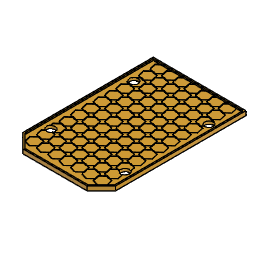
back_cover (Autodesk Fusion 360 design; units mm, degrees)
Autodesk Fusion 360 part; units mm, degrees
(part 1 of 2)
sketch "Sketch1" plane through (0, 0, 0) normal (0, 0, 1) x (1, 0, 0)
  line L0 (0, -30) -> (65.3008, -30)
  line L1 (65.3008, -30) -> (65.3008, 62.8304)
  line L2 (65.3008, 62.8304) -> (0, 62.8304)
  line L3 (0, 62.8304) -> (0, -30)
  line L4 (0, -30) -> (10, -40)
  line L5 (10, -40) -> (55.2691, -40)
  line L6 (55.2691, -40) -> (65.3008, -30)
  constraint horizontal L0
  constraint vertical L1
  constraint horizontal L2
  constraint vertical L3
  constraint perpendicular L3 L5
extrude "Extrude1" add sketch "Sketch1" against normal blind 2
sketch "Sketch2" plane through (0, 0, -2) normal (0, 0, -1) x (1, 0, 0)
  line L0 (65.3008, 30) -> (55.2691, 40)
  line L1 (55.2691, 40) -> (10, 40)
  line L2 (10, 40) -> (0, 30)
  line L3 (0, 30) -> (0, -62.8304)
  line L4 (0, -62.8304) -> (65.3008, -62.8304)
  line L5 (65.3008, -62.8304) -> (65.3008, 30)
  circle A0 centre (6.5514, 16.7159) radius 3
  circle A1 centre (6.5755, -41.7346) radius 3
  circle A2 centre (59.3355, -41.7346) radius 3
  circle A3 centre (58.8128, 16.7193) radius 3
extrude "Extrude2" cut sketch "Sketch2" against normal blind 2 contours A0 | A1 | A2 | A3
fillet "Fillet1" radius 1 3 edges at (0, 62.8304, -1) (65.3008, 62.8304, -1) (32.6504, 62.8304, 0)
sketch "Sketch3" plane through (0, 0, 0) normal (0, 0, 1) x (-1, 0, 0)
  line L0 (-65.3008, -61.8304) -> (0, -61.8304)
  line L1 (0, -61.8304) -> (0, 30)
  line L2 (0, 30) -> (-10, 40)
  line L3 (-10, 40) -> (-55.2691, 40)
  line L4 (-55.2691, 40) -> (-65.3008, 30)
  line L5 (-65.3008, 30) -> (-65.3008, -61.8304)
  circle A0 centre (-6.5514, 16.7159) radius 3
  circle A1 centre (-6.5755, -41.7346) radius 3
  circle A2 centre (-58.8128, 16.7193) radius 3
  circle A3 centre (-59.3355, -41.7346) radius 3
  line L6 (0, -61.8304) -> (0, 30)
  line L7 (0, 30) -> (-10, 40)
  line L8 (-10, 40) -> (-55.2691, 40)
  line L9 (-55.2691, 40) -> (-65.3008, 30)
  line L10 (-65.3008, 30) -> (-65.3008, -61.8304)
  line L11 (0, -61.8304) -> (-65.3008, -61.8304)
  line L12 (-1, -60.8304) -> (-1, 29.5858)
  line L13 (-1, 29.5858) -> (-10.4142, 39)
  line L14 (-10.4142, 39) -> (-54.8558, 39)
  line L15 (-54.8558, 39) -> (-64.3008, 29.5849)
  line L16 (-64.3008, 29.5849) -> (-64.3008, -60.8304)
  line L17 (-64.3008, -60.8304) -> (-1, -60.8304)
  dimension "d111" = -1
extrude "Extrude3" add sketch "Sketch3" along normal blind 1 contours L0 L1 L2 L3 L4 L5 L6 L7 L8 L9 L10 L11
sketch "Sketch4" plane through (0, 0, 0) normal (0, 0, 1) x (1, 0, 0)
  line L0 (36.6966, 8.433) -> (35.7081, 12.9448)
  line L1 (35.7081, 12.9448) -> (31.3065, 14.3446)
  line L2 (31.3065, 14.3446) -> (27.8935, 11.2327)
  line L3 (27.8935, 11.2327) -> (28.8819, 6.7209)
  line L4 (28.8819, 6.7209) -> (33.2835, 5.321)
  line L5 (33.2835, 5.321) -> (36.6966, 8.433)
  line L6 (11.7081, -27.0552) -> (7.3065, -25.6554)
  line L7 (12.6966, -31.567) -> (11.7081, -27.0552)
  line L8 (9.2835, -34.679) -> (12.6966, -31.567)
  line L9 (4.8819, -33.2791) -> (9.2835, -34.679)
  line L10 (3.8935, -28.7673) -> (4.8819, -33.2791)
  line L11 (7.3065, -25.6554) -> (3.8935, -28.7673)
  line L12 (19.7081, -27.0552) -> (15.3065, -25.6554)
  line L13 (20.6966, -31.567) -> (19.7081, -27.0552)
  line L14 (17.2835, -34.679) -> (20.6966, -31.567)
  line L15 (12.8819, -33.2791) -> (17.2835, -34.679)
  line L16 (11.8935, -28.7673) -> (12.8819, -33.2791)
  line L17 (15.3065, -25.6554) -> (11.8935, -28.7673)
  line L18 (27.7081, -27.0552) -> (23.3065, -25.6554)
  line L19 (28.6966, -31.567) -> (27.7081, -27.0552)
  line L20 (25.2835, -34.679) -> (28.6966, -31.567)
  line L21 (20.8819, -33.2791) -> (25.2835, -34.679)
  line L22 (19.8935, -28.7673) -> (20.8819, -33.2791)
  line L23 (23.3065, -25.6554) -> (19.8935, -28.7673)
  line L24 (35.7081, -27.0552) -> (31.3065, -25.6554)
  line L25 (36.6966, -31.567) -> (35.7081, -27.0552)
  line L26 (33.2835, -34.679) -> (36.6966, -31.567)
  line L27 (28.8819, -33.2791) -> (33.2835, -34.679)
  line L28 (27.8935, -28.7673) -> (28.8819, -33.2791)
  line L29 (31.3065, -25.6554) -> (27.8935, -28.7673)
  line L30 (43.7081, -27.0552) -> (39.3065, -25.6554)
  line L31 (44.6966, -31.567) -> (43.7081, -27.0552)
  line L32 (41.2835, -34.679) -> (44.6966, -31.567)
  line L33 (36.8819, -33.2791) -> (41.2835, -34.679)
  line L34 (35.8935, -28.7673) -> (36.8819, -33.2791)
  line L35 (39.3065, -25.6554) -> (35.8935, -28.7673)
  line L36 (51.7081, -27.0552) -> (47.3065, -25.6554)
  line L37 (52.6966, -31.567) -> (51.7081, -27.0552)
  line L38 (49.2835, -34.679) -> (52.6966, -31.567)
  line L39 (44.8819, -33.2791) -> (49.2835, -34.679)
  line L40 (43.8935, -28.7673) -> (44.8819, -33.2791)
  line L41 (47.3065, -25.6554) -> (43.8935, -28.7673)
  line L42 (59.7081, -27.0552) -> (55.3065, -25.6554)
  line L43 (60.6966, -31.567) -> (59.7081, -27.0552)
  line L44 (57.2835, -34.679) -> (60.6966, -31.567)
  line L45 (52.8819, -33.2791) -> (57.2835, -34.679)
  line L46 (51.8935, -28.7673) -> (52.8819, -33.2791)
  line L47 (55.3065, -25.6554) -> (51.8935, -28.7673)
  line L48 (11.7081, -19.0552) -> (7.3065, -17.6554)
  line L49 (12.6966, -23.567) -> (11.7081, -19.0552)
  line L50 (9.2835, -26.679) -> (12.6966, -23.567)
  line L51 (4.8819, -25.2791) -> (9.2835, -26.679)
  line L52 (3.8935, -20.7673) -> (4.8819, -25.2791)
  line L53 (7.3065, -17.6554) -> (3.8935, -20.7673)
  line L54 (19.7081, -19.0552) -> (15.3065, -17.6554)
  line L55 (20.6966, -23.567) -> (19.7081, -19.0552)
  line L56 (17.2835, -26.679) -> (20.6966, -23.567)
  line L57 (12.8819, -25.2791) -> (17.2835, -26.679)
  line L58 (11.8935, -20.7673) -> (12.8819, -25.2791)
  line L59 (15.3065, -17.6554) -> (11.8935, -20.7673)
  line L60 (27.7081, -19.0552) -> (23.3065, -17.6554)
  line L61 (28.6966, -23.567) -> (27.7081, -19.0552)
  line L62 (25.2835, -26.679) -> (28.6966, -23.567)
  line L63 (20.8819, -25.2791) -> (25.2835, -26.679)
  line L64 (19.8935, -20.7673) -> (20.8819, -25.2791)
  line L65 (23.3065, -17.6554) -> (19.8935, -20.7673)
  line L66 (35.7081, -19.0552) -> (31.3065, -17.6554)
  line L67 (36.6966, -23.567) -> (35.7081, -19.0552)
  line L68 (33.2835, -26.679) -> (36.6966, -23.567)
  line L69 (28.8819, -25.2791) -> (33.2835, -26.679)
  line L70 (27.8935, -20.7673) -> (28.8819, -25.2791)
  line L71 (31.3065, -17.6554) -> (27.8935, -20.7673)
  line L72 (43.7081, -19.0552) -> (39.3065, -17.6554)
  line L73 (44.6966, -23.567) -> (43.7081, -19.0552)
  line L74 (41.2835, -26.679) -> (44.6966, -23.567)
  line L75 (36.8819, -25.2791) -> (41.2835, -26.679)
  line L76 (35.8935, -20.7673) -> (36.8819, -25.2791)
  line L77 (39.3065, -17.6554) -> (35.8935, -20.7673)
  line L78 (51.7081, -19.0552) -> (47.3065, -17.6554)
  line L79 (52.6966, -23.567) -> (51.7081, -19.0552)
  line L80 (49.2835, -26.679) -> (52.6966, -23.567)
  line L81 (44.8819, -25.2791) -> (49.2835, -26.679)
  line L82 (43.8935, -20.7673) -> (44.8819, -25.2791)
  line L83 (47.3065, -17.6554) -> (43.8935, -20.7673)
  line L84 (59.7081, -19.0552) -> (55.3065, -17.6554)
  line L85 (60.6966, -23.567) -> (59.7081, -19.0552)
  line L86 (57.2835, -26.679) -> (60.6966, -23.567)
  line L87 (52.8819, -25.2791) -> (57.2835, -26.679)
  line L88 (51.8935, -20.7673) -> (52.8819, -25.2791)
  line L89 (55.3065, -17.6554) -> (51.8935, -20.7673)
  line L90 (11.7081, -11.0552) -> (7.3065, -9.6554)
  line L91 (12.6966, -15.567) -> (11.7081, -11.0552)
  line L92 (9.2835, -18.679) -> (12.6966, -15.567)
  line L93 (4.8819, -17.2791) -> (9.2835, -18.679)
  line L94 (3.8935, -12.7673) -> (4.8819, -17.2791)
  line L95 (7.3065, -9.6554) -> (3.8935, -12.7673)
  line L96 (19.7081, -11.0552) -> (15.3065, -9.6554)
  line L97 (20.6966, -15.567) -> (19.7081, -11.0552)
  line L98 (17.2835, -18.679) -> (20.6966, -15.567)
  line L99 (12.8819, -17.2791) -> (17.2835, -18.679)
  line L100 (11.8935, -12.7673) -> (12.8819, -17.2791)
  line L101 (15.3065, -9.6554) -> (11.8935, -12.7673)
  line L102 (27.7081, -11.0552) -> (23.3065, -9.6554)
  line L103 (28.6966, -15.567) -> (27.7081, -11.0552)
  line L104 (25.2835, -18.679) -> (28.6966, -15.567)
  line L105 (20.8819, -17.2791) -> (25.2835, -18.679)
  line L106 (19.8935, -12.7673) -> (20.8819, -17.2791)
  line L107 (23.3065, -9.6554) -> (19.8935, -12.7673)
  line L108 (35.7081, -11.0552) -> (31.3065, -9.6554)
  line L109 (36.6966, -15.567) -> (35.7081, -11.0552)
  line L110 (33.2835, -18.679) -> (36.6966, -15.567)
  line L111 (28.8819, -17.2791) -> (33.2835, -18.679)
  line L112 (27.8935, -12.7673) -> (28.8819, -17.2791)
  line L113 (31.3065, -9.6554) -> (27.8935, -12.7673)
  line L114 (43.7081, -11.0552) -> (39.3065, -9.6554)
  line L115 (44.6966, -15.567) -> (43.7081, -11.0552)
  line L116 (41.2835, -18.679) -> (44.6966, -15.567)
  line L117 (36.8819, -17.2791) -> (41.2835, -18.679)
  line L118 (35.8935, -12.7673) -> (36.8819, -17.2791)
  line L119 (39.3065, -9.6554) -> (35.8935, -12.7673)
  line L120 (51.7081, -11.0552) -> (47.3065, -9.6554)
  line L121 (52.6966, -15.567) -> (51.7081, -11.0552)
  line L122 (49.2835, -18.679) -> (52.6966, -15.567)
  line L123 (44.8819, -17.2791) -> (49.2835, -18.679)
  line L124 (43.8935, -12.7673) -> (44.8819, -17.2791)
  line L125 (47.3065, -9.6554) -> (43.8935, -12.7673)
  line L126 (59.7081, -11.0552) -> (55.3065, -9.6554)
  line L127 (60.6966, -15.567) -> (59.7081, -11.0552)
  line L128 (57.2835, -18.679) -> (60.6966, -15.567)
  line L129 (52.8819, -17.2791) -> (57.2835, -18.679)
  line L130 (51.8935, -12.7673) -> (52.8819, -17.2791)
  line L131 (55.3065, -9.6554) -> (51.8935, -12.7673)
  line L132 (11.7081, -3.0552) -> (7.3065, -1.6554)
  line L133 (12.6966, -7.567) -> (11.7081, -3.0552)
  line L134 (9.2835, -10.679) -> (12.6966, -7.567)
  line L135 (4.8819, -9.2791) -> (9.2835, -10.679)
  line L136 (3.8935, -4.7673) -> (4.8819, -9.2791)
  line L137 (7.3065, -1.6554) -> (3.8935, -4.7673)
  line L138 (19.7081, -3.0552) -> (15.3065, -1.6554)
  line L139 (20.6966, -7.567) -> (19.7081, -3.0552)
  line L140 (17.2835, -10.679) -> (20.6966, -7.567)
  line L141 (12.8819, -9.2791) -> (17.2835, -10.679)
  line L142 (11.8935, -4.7673) -> (12.8819, -9.2791)
  line L143 (15.3065, -1.6554) -> (11.8935, -4.7673)
  line L144 (27.7081, -3.0552) -> (23.3065, -1.6554)
  line L145 (28.6966, -7.567) -> (27.7081, -3.0552)
  line L146 (25.2835, -10.679) -> (28.6966, -7.567)
  line L147 (20.8819, -9.2791) -> (25.2835, -10.679)
  line L148 (19.8935, -4.7673) -> (20.8819, -9.2791)
  line L149 (23.3065, -1.6554) -> (19.8935, -4.7673)
  line L150 (35.7081, -3.0552) -> (31.3065, -1.6554)
  line L151 (36.6966, -7.567) -> (35.7081, -3.0552)
  line L152 (33.2835, -10.679) -> (36.6966, -7.567)
  line L153 (28.8819, -9.2791) -> (33.2835, -10.679)
  line L154 (27.8935, -4.7673) -> (28.8819, -9.2791)
  line L155 (31.3065, -1.6554) -> (27.8935, -4.7673)
  line L156 (43.7081, -3.0552) -> (39.3065, -1.6554)
  line L157 (44.6966, -7.567) -> (43.7081, -3.0552)
  line L158 (41.2835, -10.679) -> (44.6966, -7.567)
  line L159 (36.8819, -9.2791) -> (41.2835, -10.679)
  line L160 (35.8935, -4.7673) -> (36.8819, -9.2791)
  line L161 (39.3065, -1.6554) -> (35.8935, -4.7673)
  line L162 (51.7081, -3.0552) -> (47.3065, -1.6554)
  line L163 (52.6966, -7.567) -> (51.7081, -3.0552)
  line L164 (49.2835, -10.679) -> (52.6966, -7.567)
  line L165 (44.8819, -9.2791) -> (49.2835, -10.679)
  line L166 (43.8935, -4.7673) -> (44.8819, -9.2791)
  line L167 (47.3065, -1.6554) -> (43.8935, -4.7673)
  line L168 (59.7081, -3.0552) -> (55.3065, -1.6554)
  line L169 (60.6966, -7.567) -> (59.7081, -3.0552)
  line L170 (57.2835, -10.679) -> (60.6966, -7.567)
  line L171 (52.8819, -9.2791) -> (57.2835, -10.679)
  line L172 (51.8935, -4.7673) -> (52.8819, -9.2791)
  line L173 (55.3065, -1.6554) -> (51.8935, -4.7673)
  line L174 (11.7081, 4.9448) -> (7.3065, 6.3446)
  line L175 (12.6966, 0.433) -> (11.7081, 4.9448)
  line L176 (9.2835, -2.679) -> (12.6966, 0.433)
  line L177 (4.8819, -1.2791) -> (9.2835, -2.679)
  line L178 (3.8935, 3.2327) -> (4.8819, -1.2791)
  line L179 (7.3065, 6.3446) -> (3.8935, 3.2327)
  line L180 (19.7081, 4.9448) -> (15.3065, 6.3446)
  line L181 (20.6966, 0.433) -> (19.7081, 4.9448)
  line L182 (17.2835, -2.679) -> (20.6966, 0.433)
  line L183 (12.8819, -1.2791) -> (17.2835, -2.679)
  line L184 (11.8935, 3.2327) -> (12.8819, -1.2791)
  line L185 (15.3065, 6.3446) -> (11.8935, 3.2327)
  line L186 (27.7081, 4.9448) -> (23.3065, 6.3446)
  line L187 (28.6966, 0.433) -> (27.7081, 4.9448)
  line L188 (25.2835, -2.679) -> (28.6966, 0.433)
  line L189 (20.8819, -1.2791) -> (25.2835, -2.679)
  line L190 (19.8935, 3.2327) -> (20.8819, -1.2791)
  line L191 (23.3065, 6.3446) -> (19.8935, 3.2327)
  line L192 (35.7081, 4.9448) -> (31.3065, 6.3446)
  line L193 (36.6966, 0.433) -> (35.7081, 4.9448)
  line L194 (33.2835, -2.679) -> (36.6966, 0.433)
  line L195 (28.8819, -1.2791) -> (33.2835, -2.679)
  line L196 (27.8935, 3.2327) -> (28.8819, -1.2791)
  line L197 (31.3065, 6.3446) -> (27.8935, 3.2327)
  line L198 (43.7081, 4.9448) -> (39.3065, 6.3446)
  line L199 (44.6966, 0.433) -> (43.7081, 4.9448)
  line L200 (41.2835, -2.679) -> (44.6966, 0.433)
  line L201 (36.8819, -1.2791) -> (41.2835, -2.679)
  line L202 (35.8935, 3.2327) -> (36.8819, -1.2791)
  line L203 (39.3065, 6.3446) -> (35.8935, 3.2327)
  line L204 (51.7081, 4.9448) -> (47.3065, 6.3446)
  line L205 (52.6966, 0.433) -> (51.7081, 4.9448)
  line L206 (49.2835, -2.679) -> (52.6966, 0.433)
  line L207 (44.8819, -1.2791) -> (49.2835, -2.679)
  line L208 (43.8935, 3.2327) -> (44.8819, -1.2791)
  line L209 (47.3065, 6.3446) -> (43.8935, 3.2327)
  line L210 (59.7081, 4.9448) -> (55.3065, 6.3446)
  line L211 (60.6966, 0.433) -> (59.7081, 4.9448)
  line L212 (57.2835, -2.679) -> (60.6966, 0.433)
  line L213 (52.8819, -1.2791) -> (57.2835, -2.679)
  line L214 (51.8935, 3.2327) -> (52.8819, -1.2791)
  line L215 (55.3065, 6.3446) -> (51.8935, 3.2327)
  line L216 (11.7081, 12.9448) -> (7.3065, 14.3446)
  line L217 (12.6966, 8.433) -> (11.7081, 12.9448)
  line L218 (9.2835, 5.321) -> (12.6966, 8.433)
  line L219 (4.8819, 6.7209) -> (9.2835, 5.321)
  line L220 (3.8935, 11.2327) -> (4.8819, 6.7209)
  line L221 (7.3065, 14.3446) -> (3.8935, 11.2327)
  line L222 (19.7081, 12.9448) -> (15.3065, 14.3446)
  line L223 (20.6966, 8.433) -> (19.7081, 12.9448)
  line L224 (17.2835, 5.321) -> (20.6966, 8.433)
  line L225 (12.8819, 6.7209) -> (17.2835, 5.321)
  line L226 (11.8935, 11.2327) -> (12.8819, 6.7209)
  line L227 (15.3065, 14.3446) -> (11.8935, 11.2327)
  line L228 (27.7081, 12.9448) -> (23.3065, 14.3446)
  line L229 (28.6966, 8.433) -> (27.7081, 12.9448)
  line L230 (25.2835, 5.321) -> (28.6966, 8.433)
  line L231 (20.8819, 6.7209) -> (25.2835, 5.321)
  line L232 (19.8935, 11.2327) -> (20.8819, 6.7209)
  line L233 (23.3065, 14.3446) -> (19.8935, 11.2327)
  line L234 (43.7081, 12.9448) -> (39.3065, 14.3446)
  line L235 (44.6966, 8.433) -> (43.7081, 12.9448)
  line L236 (41.2835, 5.321) -> (44.6966, 8.433)
  line L237 (36.8819, 6.7209) -> (41.2835, 5.321)
  line L238 (35.8935, 11.2327) -> (36.8819, 6.7209)
  line L239 (39.3065, 14.3446) -> (35.8935, 11.2327)
  line L240 (51.7081, 12.9448) -> (47.3065, 14.3446)
  line L241 (52.6966, 8.433) -> (51.7081, 12.9448)
  line L242 (49.2835, 5.321) -> (52.6966, 8.433)
  line L243 (44.8819, 6.7209) -> (49.2835, 5.321)
  line L244 (43.8935, 11.2327) -> (44.8819, 6.7209)
  line L245 (47.3065, 14.3446) -> (43.8935, 11.2327)
  line L246 (59.7081, 12.9448) -> (55.3065, 14.3446)
  line L247 (60.6966, 8.433) -> (59.7081, 12.9448)
  line L248 (57.2835, 5.321) -> (60.6966, 8.433)
  line L249 (52.8819, 6.7209) -> (57.2835, 5.321)
  line L250 (51.8935, 11.2327) -> (52.8819, 6.7209)
  line L251 (55.3065, 14.3446) -> (51.8935, 11.2327)
  line L252 (11.7081, 20.9448) -> (7.3065, 22.3446)
  line L253 (12.6966, 16.433) -> (11.7081, 20.9448)
  line L254 (9.2835, 13.321) -> (12.6966, 16.433)
  line L255 (4.8819, 14.7209) -> (9.2835, 13.321)
  line L256 (3.8935, 19.2327) -> (4.8819, 14.7209)
  line L257 (7.3065, 22.3446) -> (3.8935, 19.2327)
  line L258 (19.7081, 20.9448) -> (15.3065, 22.3446)
  line L259 (20.6966, 16.433) -> (19.7081, 20.9448)
  line L260 (17.2835, 13.321) -> (20.6966, 16.433)
  line L261 (12.8819, 14.7209) -> (17.2835, 13.321)
  line L262 (11.8935, 19.2327) -> (12.8819, 14.7209)
  line L263 (15.3065, 22.3446) -> (11.8935, 19.2327)
  line L264 (27.7081, 20.9448) -> (23.3065, 22.3446)
  line L265 (28.6966, 16.433) -> (27.7081, 20.9448)
  line L266 (25.2835, 13.321) -> (28.6966, 16.433)
  line L267 (20.8819, 14.7209) -> (25.2835, 13.321)
  line L268 (19.8935, 19.2327) -> (20.8819, 14.7209)
  line L269 (23.3065, 22.3446) -> (19.8935, 19.2327)
  line L270 (35.7081, 20.9448) -> (31.3065, 22.3446)
  line L271 (36.6966, 16.433) -> (35.7081, 20.9448)
  line L272 (33.2835, 13.321) -> (36.6966, 16.433)
  line L273 (28.8819, 14.7209) -> (33.2835, 13.321)
  line L274 (27.8935, 19.2327) -> (28.8819, 14.7209)
  line L275 (31.3065, 22.3446) -> (27.8935, 19.2327)
  line L276 (43.7081, 20.9448) -> (39.3065, 22.3446)
  line L277 (44.6966, 16.433) -> (43.7081, 20.9448)
  line L278 (41.2835, 13.321) -> (44.6966, 16.433)
  line L279 (36.8819, 14.7209) -> (41.2835, 13.321)
  line L280 (35.8935, 19.2327) -> (36.8819, 14.7209)
  line L281 (39.3065, 22.3446) -> (35.8935, 19.2327)
  line L282 (51.7081, 20.9448) -> (47.3065, 22.3446)
  line L283 (52.6966, 16.433) -> (51.7081, 20.9448)
  line L284 (49.2835, 13.321) -> (52.6966, 16.433)
  line L285 (44.8819, 14.7209) -> (49.2835, 13.321)
  line L286 (43.8935, 19.2327) -> (44.8819, 14.7209)
  line L287 (47.3065, 22.3446) -> (43.8935, 19.2327)
  line L288 (59.7081, 20.9448) -> (55.3065, 22.3446)
  line L289 (60.6966, 16.433) -> (59.7081, 20.9448)
  line L290 (57.2835, 13.321) -> (60.6966, 16.433)
  line L291 (52.8819, 14.7209) -> (57.2835, 13.321)
  line L292 (51.8935, 19.2327) -> (52.8819, 14.7209)
  line L293 (55.3065, 22.3446) -> (51.8935, 19.2327)
  line L294 (11.7081, 28.9448) -> (7.3065, 30.3446)
  line L295 (12.6966, 24.433) -> (11.7081, 28.9448)
  line L296 (9.2835, 21.321) -> (12.6966, 24.433)
  line L297 (4.8819, 22.7209) -> (9.2835, 21.321)
  line L298 (3.8935, 27.2327) -> (4.8819, 22.7209)
  line L299 (7.3065, 30.3446) -> (3.8935, 27.2327)
  line L300 (19.7081, 28.9448) -> (15.3065, 30.3446)
  line L301 (20.6966, 24.433) -> (19.7081, 28.9448)
  line L302 (17.2835, 21.321) -> (20.6966, 24.433)
  line L303 (12.8819, 22.7209) -> (17.2835, 21.321)
  line L304 (11.8935, 27.2327) -> (12.8819, 22.7209)
  line L305 (15.3065, 30.3446) -> (11.8935, 27.2327)
  line L306 (27.7081, 28.9448) -> (23.3065, 30.3446)
  line L307 (28.6966, 24.433) -> (27.7081, 28.9448)
  line L308 (25.2835, 21.321) -> (28.6966, 24.433)
  line L309 (20.8819, 22.7209) -> (25.2835, 21.321)
  line L310 (19.8935, 27.2327) -> (20.8819, 22.7209)
  line L311 (23.3065, 30.3446) -> (19.8935, 27.2327)
  line L312 (35.7081, 28.9448) -> (31.3065, 30.3446)
  line L313 (36.6966, 24.433) -> (35.7081, 28.9448)
  line L314 (33.2835, 21.321) -> (36.6966, 24.433)
  line L315 (28.8819, 22.7209) -> (33.2835, 21.321)
  line L316 (27.8935, 27.2327) -> (28.8819, 22.7209)
  line L317 (31.3065, 30.3446) -> (27.8935, 27.2327)
  line L318 (43.7081, 28.9448) -> (39.3065, 30.3446)
  line L319 (44.6966, 24.433) -> (43.7081, 28.9448)
  line L320 (41.2835, 21.321) -> (44.6966, 24.433)
  line L321 (36.8819, 22.7209) -> (41.2835, 21.321)
  line L322 (35.8935, 27.2327) -> (36.8819, 22.7209)
  line L323 (39.3065, 30.3446) -> (35.8935, 27.2327)
  line L324 (51.7081, 28.9448) -> (47.3065, 30.3446)
  line L325 (52.6966, 24.433) -> (51.7081, 28.9448)
  line L326 (49.2835, 21.321) -> (52.6966, 24.433)
  line L327 (44.8819, 22.7209) -> (49.2835, 21.321)
  line L328 (43.8935, 27.2327) -> (44.8819, 22.7209)
  line L329 (47.3065, 30.3446) -> (43.8935, 27.2327)
  line L330 (59.7081, 28.9448) -> (55.3065, 30.3446)
  line L331 (60.6966, 24.433) -> (59.7081, 28.9448)
  line L332 (57.2835, 21.321) -> (60.6966, 24.433)
  line L333 (52.8819, 22.7209) -> (57.2835, 21.321)
  line L334 (51.8935, 27.2327) -> (52.8819, 22.7209)
  line L335 (55.3065, 30.3446) -> (51.8935, 27.2327)
  line L336 (11.7081, 36.9448) -> (7.3065, 38.3446)
  line L337 (12.6966, 32.433) -> (11.7081, 36.9448)
  line L338 (9.2835, 29.321) -> (12.6966, 32.433)
  line L339 (4.8819, 30.7209) -> (9.2835, 29.321)
  line L340 (3.8935, 35.2327) -> (4.8819, 30.7209)
  line L341 (7.3065, 38.3446) -> (3.8935, 35.2327)
  line L342 (19.7081, 36.9448) -> (15.3065, 38.3446)
  line L343 (20.6966, 32.433) -> (19.7081, 36.9448)
  line L344 (17.2835, 29.321) -> (20.6966, 32.433)
  line L345 (12.8819, 30.7209) -> (17.2835, 29.321)
  line L346 (11.8935, 35.2327) -> (12.8819, 30.7209)
  line L347 (15.3065, 38.3446) -> (11.8935, 35.2327)
  line L348 (27.7081, 36.9448) -> (23.3065, 38.3446)
  line L349 (28.6966, 32.433) -> (27.7081, 36.9448)
  line L350 (25.2835, 29.321) -> (28.6966, 32.433)
  line L351 (20.8819, 30.7209) -> (25.2835, 29.321)
  line L352 (19.8935, 35.2327) -> (20.8819, 30.7209)
  line L353 (23.3065, 38.3446) -> (19.8935, 35.2327)
  line L354 (35.7081, 36.9448) -> (31.3065, 38.3446)
  line L355 (36.6966, 32.433) -> (35.7081, 36.9448)
  line L356 (33.2835, 29.321) -> (36.6966, 32.433)
  line L357 (28.8819, 30.7209) -> (33.2835, 29.321)
  line L358 (27.8935, 35.2327) -> (28.8819, 30.7209)
  line L359 (31.3065, 38.3446) -> (27.8935, 35.2327)
  line L360 (43.7081, 36.9448) -> (39.3065, 38.3446)
  line L361 (44.6966, 32.433) -> (43.7081, 36.9448)
  line L362 (41.2835, 29.321) -> (44.6966, 32.433)
  line L363 (36.8819, 30.7209) -> (41.2835, 29.321)
  line L364 (35.8935, 35.2327) -> (36.8819, 30.7209)
  line L365 (39.3065, 38.3446) -> (35.8935, 35.2327)
  line L366 (51.7081, 36.9448) -> (47.3065, 38.3446)
  line L367 (52.6966, 32.433) -> (51.7081, 36.9448)
  line L368 (49.2835, 29.321) -> (52.6966, 32.433)
  line L369 (44.8819, 30.7209) -> (49.2835, 29.321)
  line L370 (43.8935, 35.2327) -> (44.8819, 30.7209)
  line L371 (47.3065, 38.3446) -> (43.8935, 35.2327)
  line L372 (59.7081, 36.9448) -> (55.3065, 38.3446)
  line L373 (60.6966, 32.433) -> (59.7081, 36.9448)
  line L374 (57.2835, 29.321) -> (60.6966, 32.433)
  line L375 (52.8819, 30.7209) -> (57.2835, 29.321)
  line L376 (51.8935, 35.2327) -> (52.8819, 30.7209)
  line L377 (55.3065, 38.3446) -> (51.8935, 35.2327)
  line L378 (11.7081, 44.9448) -> (7.3065, 46.3446)
  line L379 (12.6966, 40.433) -> (11.7081, 44.9448)
  line L380 (9.2835, 37.321) -> (12.6966, 40.433)
  line L381 (4.8819, 38.7209) -> (9.2835, 37.321)
  line L382 (3.8935, 43.2327) -> (4.8819, 38.7209)
  line L383 (7.3065, 46.3446) -> (3.8935, 43.2327)
  line L384 (19.7081, 44.9448) -> (15.3065, 46.3446)
  line L385 (20.6966, 40.433) -> (19.7081, 44.9448)
  line L386 (17.2835, 37.321) -> (20.6966, 40.433)
  line L387 (12.8819, 38.7209) -> (17.2835, 37.321)
  line L388 (11.8935, 43.2327) -> (12.8819, 38.7209)
  line L389 (15.3065, 46.3446) -> (11.8935, 43.2327)
  line L390 (27.7081, 44.9448) -> (23.3065, 46.3446)
  line L391 (28.6966, 40.433) -> (27.7081, 44.9448)
  line L392 (25.2835, 37.321) -> (28.6966, 40.433)
  line L393 (20.8819, 38.7209) -> (25.2835, 37.321)
  line L394 (19.8935, 43.2327) -> (20.8819, 38.7209)
  line L395 (23.3065, 46.3446) -> (19.8935, 43.2327)
  line L396 (35.7081, 44.9448) -> (31.3065, 46.3446)
  line L397 (36.6966, 40.433) -> (35.7081, 44.9448)
  line L398 (33.2835, 37.321) -> (36.6966, 40.433)
  line L399 (28.8819, 38.7209) -> (33.2835, 37.321)
  line L400 (27.8935, 43.2327) -> (28.8819, 38.7209)
  line L401 (31.3065, 46.3446) -> (27.8935, 43.2327)
  line L402 (43.7081, 44.9448) -> (39.3065, 46.3446)
  line L403 (44.6966, 40.433) -> (43.7081, 44.9448)
  line L404 (41.2835, 37.321) -> (44.6966, 40.433)
  line L405 (36.8819, 38.7209) -> (41.2835, 37.321)
  line L406 (35.8935, 43.2327) -> (36.8819, 38.7209)
  line L407 (39.3065, 46.3446) -> (35.8935, 43.2327)
  line L408 (51.7081, 44.9448) -> (47.3065, 46.3446)
  line L409 (52.6966, 40.433) -> (51.7081, 44.9448)
  line L410 (49.2835, 37.321) -> (52.6966, 40.433)
  line L411 (44.8819, 38.7209) -> (49.2835, 37.321)
  line L412 (43.8935, 43.2327) -> (44.8819, 38.7209)
  line L413 (47.3065, 46.3446) -> (43.8935, 43.2327)
  line L414 (59.7081, 44.9448) -> (55.3065, 46.3446)
  line L415 (60.6966, 40.433) -> (59.7081, 44.9448)
  line L416 (57.2835, 37.321) -> (60.6966, 40.433)
  line L417 (52.8819, 38.7209) -> (57.2835, 37.321)
  line L418 (51.8935, 43.2327) -> (52.8819, 38.7209)
  line L419 (55.3065, 46.3446) -> (51.8935, 43.2327)
  line L420 (11.7081, 52.9448) -> (7.3065, 54.3446)
  line L421 (12.6966, 48.433) -> (11.7081, 52.9448)
  line L422 (9.2835, 45.321) -> (12.6966, 48.433)
  line L423 (4.8819, 46.7209) -> (9.2835, 45.321)
  line L424 (3.8935, 51.2327) -> (4.8819, 46.7209)
  line L425 (7.3065, 54.3446) -> (3.8935, 51.2327)
  line L426 (19.7081, 52.9448) -> (15.3065, 54.3446)
  line L427 (20.6966, 48.433) -> (19.7081, 52.9448)
  line L428 (17.2835, 45.321) -> (20.6966, 48.433)
  line L429 (12.8819, 46.7209) -> (17.2835, 45.321)
  line L430 (11.8935, 51.2327) -> (12.8819, 46.7209)
  line L431 (15.3065, 54.3446) -> (11.8935, 51.2327)
  line L432 (27.7081, 52.9448) -> (23.3065, 54.3446)
  line L433 (28.6966, 48.433) -> (27.7081, 52.9448)
  line L434 (25.2835, 45.321) -> (28.6966, 48.433)
  line L435 (20.8819, 46.7209) -> (25.2835, 45.321)
  line L436 (19.8935, 51.2327) -> (20.8819, 46.7209)
  line L437 (23.3065, 54.3446) -> (19.8935, 51.2327)
  line L438 (35.7081, 52.9448) -> (31.3065, 54.3446)
  line L439 (36.6966, 48.433) -> (35.7081, 52.9448)
  line L440 (33.2835, 45.321) -> (36.6966, 48.433)
  line L441 (28.8819, 46.7209) -> (33.2835, 45.321)
  line L442 (27.8935, 51.2327) -> (28.8819, 46.7209)
  line L443 (31.3065, 54.3446) -> (27.8935, 51.2327)
  line L444 (43.7081, 52.9448) -> (39.3065, 54.3446)
  line L445 (44.6966, 48.433) -> (43.7081, 52.9448)
  line L446 (41.2835, 45.321) -> (44.6966, 48.433)
  line L447 (36.8819, 46.7209) -> (41.2835, 45.321)
  line L448 (35.8935, 51.2327) -> (36.8819, 46.7209)
  line L449 (39.3065, 54.3446) -> (35.8935, 51.2327)
  line L450 (51.7081, 52.9448) -> (47.3065, 54.3446)
  line L451 (52.6966, 48.433) -> (51.7081, 52.9448)
  line L452 (49.2835, 45.321) -> (52.6966, 48.433)
  line L453 (44.8819, 46.7209) -> (49.2835, 45.321)
  line L454 (43.8935, 51.2327) -> (44.8819, 46.7209)
  line L455 (47.3065, 54.3446) -> (43.8935, 51.2327)
  line L456 (59.7081, 52.9448) -> (55.3065, 54.3446)
  line L457 (60.6966, 48.433) -> (59.7081, 52.9448)
  line L458 (57.2835, 45.321) -> (60.6966, 48.433)
  line L459 (52.8819, 46.7209) -> (57.2835, 45.321)
  line L460 (51.8935, 51.2327) -> (52.8819, 46.7209)
  line L461 (55.3065, 54.3446) -> (51.8935, 51.2327)
  line L462 (11.7081, 60.9448) -> (7.3065, 62.3446)
  line L463 (12.6966, 56.433) -> (11.7081, 60.9448)
  line L464 (9.2835, 53.321) -> (12.6966, 56.433)
  line L465 (4.8819, 54.7209) -> (9.2835, 53.321)
  line L466 (3.8935, 59.2327) -> (4.8819, 54.7209)
  line L467 (7.3065, 62.3446) -> (3.8935, 59.2327)
  line L468 (19.7081, 60.9448) -> (15.3065, 62.3446)
  line L469 (20.6966, 56.433) -> (19.7081, 60.9448)
  line L470 (17.2835, 53.321) -> (20.6966, 56.433)
  line L471 (12.8819, 54.7209) -> (17.2835, 53.321)
  line L472 (11.8935, 59.2327) -> (12.8819, 54.7209)
  line L473 (15.3065, 62.3446) -> (11.8935, 59.2327)
  line L474 (27.7081, 60.9448) -> (23.3065, 62.3446)
  line L475 (28.6966, 56.433) -> (27.7081, 60.9448)
  line L476 (25.2835, 53.321) -> (28.6966, 56.433)
  line L477 (20.8819, 54.7209) -> (25.2835, 53.321)
  line L478 (19.8935, 59.2327) -> (20.8819, 54.7209)
  line L479 (23.3065, 62.3446) -> (19.8935, 59.2327)
  line L480 (35.7081, 60.9448) -> (31.3065, 62.3446)
  line L481 (36.6966, 56.433) -> (35.7081, 60.9448)
  line L482 (33.2835, 53.321) -> (36.6966, 56.433)
  line L483 (28.8819, 54.7209) -> (33.2835, 53.321)
  line L484 (27.8935, 59.2327) -> (28.8819, 54.7209)
  line L485 (31.3065, 62.3446) -> (27.8935, 59.2327)
  line L486 (43.7081, 60.9448) -> (39.3065, 62.3446)
  line L487 (44.6966, 56.433) -> (43.7081, 60.9448)
  line L488 (41.2835, 53.321) -> (44.6966, 56.433)
  line L489 (36.8819, 54.7209) -> (41.2835, 53.321)
  line L490 (35.8935, 59.2327) -> (36.8819, 54.7209)
  line L491 (39.3065, 62.3446) -> (35.8935, 59.2327)
  line L492 (51.7081, 60.9448) -> (47.3065, 62.3446)
  line L493 (52.6966, 56.433) -> (51.7081, 60.9448)
  line L494 (49.2835, 53.321) -> (52.6966, 56.433)
  line L495 (44.8819, 54.7209) -> (49.2835, 53.321)
  line L496 (43.8935, 59.2327) -> (44.8819, 54.7209)
  line L497 (47.3065, 62.3446) -> (43.8935, 59.2327)
  line L498 (59.7081, 60.9448) -> (55.3065, 62.3446)
  line L499 (60.6966, 56.433) -> (59.7081, 60.9448)
  line L500 (57.2835, 53.321) -> (60.6966, 56.433)
  line L501 (52.8819, 54.7209) -> (57.2835, 53.321)
  line L502 (51.8935, 59.2327) -> (52.8819, 54.7209)
  line L503 (55.3065, 62.3446) -> (51.8935, 59.2327)
  point P0 (32.295, 9.8328)
  dimension "d123" = 4
  dimension "d126" = 8
  dimension "d127" = 8
  measures "d123" distance of P0 L5
extrude "Extrude4" cut sketch "Sketch4" against normal blind 0.3 contours L0 L5 L198 L203 L234 L235 L236 L237 L238 L239 L244 L245 L278 L279 | L0 L1 L2 L3 L4 L5 L192 L197 L229 L230 L238 L239 L272 L273 | L234 L239 L271 L272 L276 L277 L278 L279 L280 L281 L286 L287 L320 L321 | L4 L5 L150 L155 L187 L188 L192 L193 L194 L195 L196 L197 L202 L203 | L1 L2 L265 L266 L270 L271 L272 L273 L274 L275 L280 L281 L314 L315 | L156 L161 L193 L194 L198 L199 L200 L201 L202 L203 L208 L209 L236 L237 | L240 L245 L277 L278 L282 L283 L284 L285 L286 L287 L292 L293 L326 L327 | L144 L149 L181 L182 L186 L187 L188 L189 L190 L191 L196 L197 L230 L231 | L2 L3 L186 L191 L223 L224 L228 L229 L230 L231 L232 L233 L266 L267 | L204 L209 L235 L236 L240 L241 L242 L243 L244 L245 L250 L251 L284 L285 | L228 L233 L259 L260 L264 L265 L266 L267 L268 L269 L274 L275 L308 L309 | L276 L281 L313 L314 L318 L319 L320 L321 L322 L323 L328 L329 L362 L363 | L108 L113 L145 L146 L150 L151 L152 L153 L154 L155 L160 L161 L194 L195 | L162 L167 L199 L200 L204 L205 L206 L207 L208 L209 L214 L215 L242 L243 | L270 L275 L307 L308 L312 L313 L314 L315 L316 L317 L322 L323 L356 L357 | L282 L287 L319 L320 L324 L325 L326 L327 L328 L329 L334 L335 L368 L369 | L102 L107 L139 L140 L144 L145 L146 L147 L148 L149 L154 L155 L188 L189 | L114 L119 L151 L152 L156 L157 L158 L159 L160 L161 L166 L167 L200 L201 | L246 L251 L283 L284 L288 L289 L290 L291 L292 L293 L332 L333 | L138 L143 L175 L176 L180 L181 L182 L183 L184 L185 L190 L191 L224 L225 | L180 L185 L217 L218 L222 L223 L224 L225 L226 L227 L232 L233 L260 L261 | L264 L269 L301 L302 L306 L307 L308 L309 L310 L311 L316 L317 L350 L351 | L210 L215 L241 L242 L246 L247 L248 L249 L250 L251 L290 L291 | L288 L293 L325 L326 L330 L331 L332 L333 L334 L335 L374 L375 | L96 L101 L133 L134 L138 L139 L140 L141 L142 L143 L148 L149 L182 L183 | L120 L125 L157 L158 L162 L163 L164 L165 L166 L167 L172 L173 L206 L207 | L222 L227 L253 L254 L258 L259 L260 L261 L262 L263 L268 L269 L302 L303 | L318 L323 L355 L356 L360 L361 L362 L363 L364 L365 L370 L371 L404 L405 | L66 L71 L103 L104 L108 L109 L110 L111 L112 L113 L118 L119 L152 L153 | L168 L173 L205 L206 L210 L211 L212 L213 L214 L215 L248 L249 | L312 L317 L349 L350 L354 L355 L356 L357 L358 L359 L364 L365 L398 L399 | L324 L329 L361 L362 L366 L367 L368 L369 L370 L371 L376 L377 L410 L411 | L60 L65 L97 L98 L102 L103 L104 L105 L106 L107 L112 L113 L146 L147 | L72 L77 L109 L110 L114 L115 L116 L117 L118 L119 L124 L125 L158 L159 | L330 L335 L367 L368 L372 L373 L374 L375 L376 L377 L416 L417 | L54 L59 L91 L92 L96 L97 L98 L99 L100 L101 L106 L107 L140 L141 | L258 L263 L295 L296 L300 L301 L302 L303 L304 L305 L310 L311 L344 L345 | L132 L137 L174 L175 L176 L177 L178 L179 L184 L185 L218 L219 | L126 L131 L163 L164 L168 L169 L170 L171 L172 L173 L212 L213 | L174 L179 L216 L217 L218 L219 L220 L221 L226 L227 L254 L255 | L306 L311 L343 L344 L348 L349 L350 L351 L352 L353 L358 L359 L392 L393 | L90 L95 L132 L133 L134 L135 L136 L137 L142 L143 L176 L177 | L78 L83 L115 L116 L120 L121 L122 L123 L124 L125 L130 L131 L164 L165 | L216 L221 L252 L253 L254 L255 L256 L257 L262 L263 L296 L297 | L360 L365 L397 L398 L402 L403 L404 L405 L406 L407 L412 L413 L446 L447 | L48 L53 L90 L91 L92 L93 L94 L95 L100 L101 L134 L135 | L24 L29 L61 L62 L66 L67 L68 L69 L70 L71 L76 L77 L110 L111 | L354 L359 L391 L392 L396 L397 L398 L399 L400 L401 L406 L407 L440 L441 | L366 L371 L403 L404 L408 L409 L410 L411 L412 L413 L418 L419 L452 L453 | L18 L23 L55 L56 L60 L61 L62 L63 L64 L65 L70 L71 L104 L105 | L30 L35 L67 L68 L72 L73 L74 L75 L76 L77 L82 L83 L116 L117 | L300 L305 L337 L338 L342 L343 L344 L345 L346 L347 L352 L353 L386 L387 | L372 L377 L409 L410 L414 L415 L416 L417 L418 L419 L458 L459 | L12 L17 L49 L50 L54 L55 L56 L57 L58 L59 L64 L65 L98 L99 | L84 L89 L121 L122 L126 L127 L128 L129 L130 L131 L170 L171 | L252 L257 L294 L295 L296 L297 L298 L299 L304 L305 L338 L339 | L6 L11 L48 L49 L50 L51 L52 L53 L58 L59 L92 L93 | L348 L353 L385 L386 L390 L391 L392 L393 L394 L395 L400 L401 L434 L435 | L36 L41 L73 L74 L78 L79 L80 L81 L82 L83 L88 L89 L122 L123 | L402 L407 L439 L440 L444 L445 L446 L447 L448 L449 L454 L455 L488 L489 | L414 L419 L451 L452 L456 L457 L458 L459 L460 L461 L500 L501 | L19 L20 L24 L25 L26 L27 L28 L29 L34 L35 L68 L69 | L294 L299 L336 L337 L338 L339 L340 L341 L346 L347 L380 L381 | L396 L401 L433 L434 L438 L439 L440 L441 L442 L443 L448 L449 L482 L483 | L408 L413 L445 L446 L450 L451 L452 L453 L454 L455 L460 L461 L494 L495 | L13 L14 L18 L19 L20 L21 L22 L23 L28 L29 L62 L63 | L25 L26 L30 L31 L32 L33 L34 L35 L40 L41 L74 L75 | L342 L347 L379 L380 L384 L385 L386 L387 L388 L389 L394 L395 L428 L429 | L7 L8 L12 L13 L14 L15 L16 L17 L22 L23 L56 L57 | L42 L47 L79 L80 L84 L85 L86 L87 L88 L89 L128 L129 | L456 L461 L493 L494 L498 L499 L500 L501 L502 L503 | L6 L7 L8 L9 L10 L11 L16 L17 L50 L51 | L390 L395 L427 L428 L432 L433 L434 L435 L436 L437 L442 L443 L476 L477 | L31 L32 L36 L37 L38 L39 L40 L41 L46 L47 L80 L81 | L336 L341 L378 L379 L380 L381 L382 L383 L388 L389 L422 L423 | L444 L449 L481 L482 L486 L487 L488 L489 L490 L491 L496 L497 | L37 L38 L42 L43 L44 L45 L46 L47 L86 L87 | L438 L443 L475 L476 L480 L481 L482 L483 L484 L485 L490 L491 | L450 L455 L487 L488 L492 L493 L494 L495 L496 L497 L502 L503 | L384 L389 L421 L422 L426 L427 L428 L429 L430 L431 L436 L437 L470 L471 | L432 L437 L469 L470 L474 L475 L476 L477 L478 L479 L484 L485 | L378 L383 L420 L421 L422 L423 L424 L425 L430 L431 L464 L465 | L426 L431 L463 L464 L468 L469 L470 L471 L472 L473 L478 L479 | L420 L425 L462 L463 L464 L465 L466 L467 L472 L473